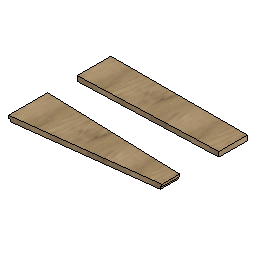
Ramps (Autodesk Fusion 360 design; units mm, degrees)
Autodesk Fusion 360 part; units mm, degrees
sketch "Skizze1" plane through (0, 0, 0) normal (0, 0, 1) x (1, 0, 0)
  line L0 (0, 0) -> (0, 171)
  line L1 (0, 171) -> (694, 171)
  line L2 (694, 171) -> (694, 26)
  line L3 (694, 26) -> (0, 0)
  line L4 (0, -150) -> (0, -348.87)
  line L5 (0, -150) -> (693.6184, -173.0097)
  line L6 (693.6184, -173.0097) -> (693.6184, -263.0197)
  line L7 (693.6184, -263.0197) -> (0, -348.87)
  dimension "d1" = 171
  dimension "d2" = 145
  dimension "d3" = 694
  dimension "d4" = 198.87
  dimension "d5" = 694
  dimension "d6" = 88.1
  dimension "d7" = 90.01
  dimension "d8" = 91.9
  dimension "d9" = 150
  constraint vertical L0
  constraint perpendicular L0 L1
  constraint perpendicular L1 L2
  constraint coincident L0.start L3.end
  constraint parallel L0 L4
  constraint collinear L0 L4
  measures "d1" distance of L0.start L0.end
  measures "d2" distance of L1.end L2.end
  measures "d3" distance of L0.end L1.end
  measures "d4" distance of L4.start L4.end
  measures "d5" distance of L4.start L5.end
  measures "d6" angle of L4 L5
  measures "d7" distance of L5.end L6.end
  measures "d8" angle of L5 L6
  measures "d9" distance of L0.start L4.start
extrude "Extrusion1" add sketch "Skizze1" along normal blind 25 makes body 1 at (231.2061, -253.9632, 0) makes body 2 at (231.3333, 65.6667, 0)
copy_body "Körper->Berechn1" bodies 1 removing the originals makes body 3 in component "Boden"
copy_body "Körper->Berechn2" bodies 2 removing the originals makes body 4 in component "Innenwand"
sketch "Skizze1 (2)" plane through (0, 0, 0) normal (0, 0, -1) x (1, 0, 0) in component "Boden"
  line L0 (0, 348.87) -> (0, 150)
  line L1 (0, 150) -> (693.6184, 173.0097)
  line L2 (693.6184, 173.0097) -> (693.6184, 263.0197)
  line L3 (693.6184, 263.0197) -> (0, 348.87)
  line L4 (8, 347.8798) -> (8, 150.2654)
  line L5 (686.6184, 263.8861) -> (686.6184, 172.7775)
  dimension "d12" = 8
  dimension "d13" = 7
  constraint coincident L3 L4.start
  constraint coincident L1 L4.end
  constraint parallel L0 L4
  constraint coincident L3 L5.start
  constraint coincident L1 L5.end
  constraint parallel L2 L5
  measures "d12" distance of L0 L4
  measures "d13" distance of L2 L5
extrude "Extrusion1'" cut sketch "Skizze1 (2)" against normal blind 14 contours L1 L2 L3 L5 bodies 3 in component "Boden"
extrude "Extrusion2" cut sketch "Skizze1 (2)" against normal blind 11 contours L0 L1 L3 L4 bodies 3 in component "Boden"
component "Boden" placed x (1, 0, 0) y (0, 1, 0) z (0, 0, 1) at (0, 0, 0)
component "Innenwand" placed x (1, 0, 0) y (0, 1, 0) z (0, 0, 1) at (0, 0, 0)
